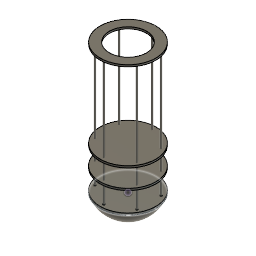
cansat+body (Autodesk Fusion 360 archive; units mm, degrees)
design "cansat body"
Autodesk Fusion 360 part; units mm, degrees
sketch "Sketch1" plane through (0, 0, 0) normal (0, 1, 0) x (1, 0, 0)
  circle A0 centre (0, 0) radius 75
  dimension "d1" = 150
  constraint coincident A0.centre origin
  measures "d1" diameter of A0
extrude "Extrude1" add sketch "Sketch1" along normal blind 5 makes body 1
sketch "Sketch2" plane through (0, 5, 0) normal (0, 1, 0) x (-1, 0, 0)
  circle A0 centre (0, 0) radius 75
  circle A1 centre (0.0043, -65) radius 2.5
  circle A2 centre (56.2938, -32.4963) radius 2.5
  circle A3 centre (56.2895, 32.5037) radius 2.5
  circle A4 centre (-56.2895, -32.5037) radius 2.5
  circle A5 centre (-0.0043, 65) radius 2.5
  circle A6 centre (-56.2938, 32.4963) radius 2.5
  dimension "d4" = 65
  dimension "d5" = 5
  dimension "d6" = 5
  dimension "d7" = 5
  dimension "d8" = 5
  dimension "d9" = 5
  dimension "d10" = 5
  constraint coincident A0.centre origin
  measures "d4" distance of A0.centre A5.centre
  measures "d5" diameter of A1
  measures "d6" diameter of A2
  measures "d7" diameter of A3
  measures "d8" diameter of A4
  measures "d9" diameter of A5
  measures "d10" diameter of A6
extrude "Extrude2" add sketch "Sketch2" along normal blind 350 contours A1 | A2 | A3 | A4 | A5 | A6 bodies 1
ref_plane "WorkPlane1" through (0, 355, 0) normal (0, 1, 0) x (1, 0, 0)
sketch "Sketch3" plane through (0, 355, 0) normal (0, 1, 0) x (1, 0, 0)
  circle A0 centre (0, 0) radius 75
  dimension "d14" = 150
  constraint coincident A0.centre origin
  measures "d14" diameter of A0
extrude "Extrude3" cut sketch "Sketch3" against normal blind 5 bodies 1
extrude "Extrude4" add sketch "Sketch3" against normal blind 5 from surface at -5 bodies 1
sketch "Sketch4" plane through (0, 350, 0) normal (0, 1, 0) x (-1, 0, 0)
  circle A0 centre (0, 0) radius 75
  circle A1 centre (0, 0) radius 50
  dimension "d19" = 100
  constraint coincident A0.centre A1.centre
  measures "d19" diameter of A1
extrude "Extrude5" cut sketch "Sketch4" against normal blind 5 contours A1 bodies 1
ref_plane "WorkPlane2" through (0, 110, 0) normal (0, 1, 0) x (1, 0, 0)
ref_plane "WorkPlane3" through (0, 57.5, 0) normal (0, 1, 0) x (1, 0, 0)
sketch "Sketch5" plane through (0, 110, 0) normal (0, 1, 0) x (1, 0, 0)
  circle A0 centre (0, 0) radius 75
  dimension "d24" = 150
  constraint coincident A0.centre origin
  measures "d24" diameter of A0
sketch "Sketch6" plane through (0, 57.5, 0) normal (0, 1, 0) x (1, 0, 0)
  circle A0 centre (0, 0) radius 75
  dimension "d25" = 150
  constraint coincident A0.centre origin
  measures "d25" diameter of A0
extrude "Extrude6" add sketch "Sketch5" along normal blind 5 separate body makes body 2
extrude "Extrude7" add sketch "Sketch6" along normal blind 5 separate body makes body 3
ref_plane "WorkPlane4" through (0, 2.5, 0) normal (0, 0, 1) x (0, 1, 0)
sketch "Sketch7" plane through (0, 0, 0) normal (0, 0, 1) x (1, 0, 0)
  line L0 (0, 0) -> (0, -50)
  arc A0 (0, -50) -> (75, 0) centre (3.5, 26) ccw
  line L1 (0, 0) -> (75, 0)
  dimension "d31" = 50
  constraint coincident L0.start L1.start
  constraint vertical L0
  constraint perpendicular L0 L1
  measures "d31" distance of L0.start L0.end
revolve "Revolve1" add sketch "Sketch7" angle 360 about axis through (0, 0, 0) along (0, -1, 0) bodies 1

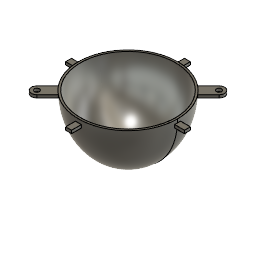
design "parachute container"
Autodesk Fusion 360 part; units mm, degrees
sketch "Sketch1" plane through (0, 0, 0) normal (0, 0, 1) x (1, 0, 0)
  line L0 (48, 0) -> (50, 0)
  ellipse E0 centre (0, 0) end of major axis (0, -60) minor radius 50 (0, -60) -> (50, 0) ccw
  line L1 (0, 0) -> (0, -38) construction
  spline S0 degree 3 poles (0, -58) (7.8191, -58) (15.6371, -55.6479) (22.5715, -51.1795) (29.3821, -46.7908) (35.3239, -40.3623) (39.6928, -32.5994) (44.1366, -24.7033) (46.9393, -15.4428) (47.7489, -5.9208) (47.9162, -3.9542) (48, -1.9771) (48, 0) knots 0 0 0 0 0.492802 0.492802 0.492802 0.976806 0.976806 0.976806 1.469118 1.469118 1.469118 1.570796 1.570796 1.570796 1.570796
  line L2 (0, -58) -> (0, -60)
  line L3 (0, -61.952) -> (0, -64)
  line L4 (0, -66) -> (2, -66)
  line L5 (2, -66) -> (2, -59.952)
  line L6 (0, -60) -> (-4, -60)
  line L7 (-4, -60) -> (-4, -66)
  line L8 (-4, -66) -> (0, -66)
  line L9 (-2, -61.952) -> (-2, -64)
  line L10 (-2, -61.952) -> (0, -61.952)
  line L11 (-2, -64) -> (0, -64)
  dimension "d1" = 120
  dimension "d2" = 100
  dimension "d12" = 6
  dimension "d13" = 2
  dimension "d14" = 4
  dimension "d16" = 2
  dimension "d18" = 2
  constraint coincident E0.centre L1.start
  constraint vertical L2
  constraint parallel L2 L3
  constraint perpendicular L3 L4
  constraint perpendicular L4 L5
  constraint coincident E0 L5.end
  constraint tangent E0 L6
  constraint perpendicular L2 L6
  constraint perpendicular L6 L7
  constraint perpendicular L8 L9
  constraint perpendicular L5 L10
  constraint perpendicular L5 L11
  measures "d1" distance of E0
  measures "d12" distance of L2.end L4.start
  measures "d13" distance of L4.start L4.end
  measures "d14" distance of L2.end L6.end
  measures "d16" distance of L7 L9
  measures "d18" distance of L4 L11
revolve "Revolve2" add sketch "Sketch1" angle 360 about axis through (0, 1.75, 0) along (0, 1, 0) contours L0 E0 S0 L2 makes body 1
extrude "Extrude1" add sketch "Sketch1" along normal mid plane 4 separate body contours E0 L4 L5 L6 L7 L8 makes body 2
sketch "Sketch2" plane through (0, 0, 0) normal (0, 0, 1) x (1, 0, 0)
  line L0 (3, -6.5) -> (-3, -6.5)
  line L1 (-3, -6.5) -> (-3, -3.5)
  line L2 (-3, -3.5) -> (3, -3.5)
  line L3 (3, -3.5) -> (3, -6.5)
  line L4 (3, -6.5) -> (-3, -3.5) construction
  line L5 (-3, -6.5) -> (3, -3.5) construction
  point P0 (0, -5)
  dimension "d40" = 6
  dimension "d41" = 3
  dimension "d42" = 5
  constraint horizontal L0
  constraint perpendicular L0 L1
  constraint parallel L0 L2
  constraint parallel L1 L3
  constraint coincident L4 P0
  constraint coincident L5 P0
  measures "d40" distance of L1.end L2.end
  measures "d41" distance of L0.end L1.end
  measures "d42" distance of origin P0
extrude "Extrude2" add sketch "Sketch2" along normal blind 10 from surface at 50 separate body makes body 3
pattern_circular "C-Pattern1" count 4 over 360 about axis through (0, 1.75, 0) along (0, 1, 0) of "Extrude2" makes body 4 at (53.3333, -6.5, -1) makes body 5 at (-1, -6.5, -53.3333) makes body 6 at (-53.3333, -6.5, 1)
sketch "Sketch3" plane through (0, 0, 0) normal (0, 1, 0) x (1, 0, 0)
  line L0 (0, 0) -> (57.0088, 0) construction
  circle A0 centre (45.9619, 45.9619) radius 2.55
  arc A1 (39.0613, 31.2124) -> (31.1808, 39.0865) centre (0, 0) ccw
  line L1 (42.0478, 49.8967) -> (31.1808, 39.0865)
  line L2 (49.8864, 42.0375) -> (39.0613, 31.2124)
  arc A2 (49.8864, 42.0375) -> (42.0478, 49.8967) centre (45.9619, 45.9619) ccw
  line L3 (0, 0) -> (-42.4264, 42.4264) construction
  line L4 (0, 0) -> (60, 0) construction
  line L5 (-49.8967, -42.0478) -> (-39.0865, -31.1808)
  arc A3 (-39.0865, -31.1808) -> (-31.2124, -39.0613) centre (0, 0) ccw
  line L6 (-42.0375, -49.8864) -> (-31.2124, -39.0613)
  circle A4 centre (-45.9619, -45.9619) radius 2.55
  arc A5 (-49.8967, -42.0478) -> (-42.0375, -49.8864) centre (-45.9619, -45.9619) ccw
  dimension "d29" = 65
  dimension "d30" = 5.1
  dimension "d31" = 100
  dimension "d36" = 135
  constraint horizontal L0
  constraint coincident L0.start A1.centre
  constraint concentric A0 A2
  constraint horizontal L4
  constraint symmetric A0 L3 A4
  constraint symmetric A1 L3 A3
  constraint symmetric L1.start L3 L5.start
  constraint symmetric L2.start L3 L6.start
  constraint symmetric A1.end L3 L5.end
  constraint symmetric A1.start L3 A3.end
  constraint symmetric A2 L3 A5
  measures "d29" distance of L0.start A0.centre
  measures "d30" diameter of A0
  measures "d31" diameter of A1
  measures "d36" angle of L3 L4
extrude "Extrude3" add sketch "Sketch3" against normal blind 3 bodies 1 2

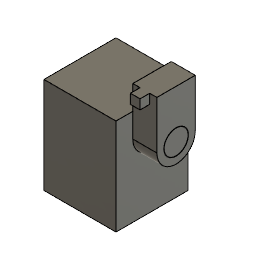
design "motor"
Autodesk Fusion 360 part; units mm, degrees
sketch "Sketch1" plane through (0, 0, 0) normal (0, 1, 0) x (1, 0, 0)
  line L0 (7.5, 7.5) -> (-7.5, 7.5)
  line L1 (-7.5, 7.5) -> (-7.5, -7.5)
  line L2 (-7.5, -7.5) -> (7.5, -7.5)
  line L3 (7.5, -7.5) -> (7.5, 7.5)
  line L4 (7.5, 7.5) -> (-7.5, -7.5) construction
  line L5 (-7.5, 7.5) -> (7.5, -7.5) construction
  dimension "d1" = 15
  dimension "d2" = 15
  constraint horizontal L0
  constraint perpendicular L0 L1
  constraint parallel L0 L2
  constraint parallel L1 L3
  constraint coincident L4 origin
  constraint coincident L5 origin
  measures "d1" distance of L1.end L2.end
  measures "d2" distance of L0.end L1.end
extrude "Extrude1" add sketch "Sketch1" along normal blind 20
sketch "Sketch2" plane through (7.5, 0, 0) normal (1, 0, 0) x (0, 0, -1)
  line L0 (-7.5, 0) -> (7.5, 0)
  line L1 (7.5, 0) -> (7.5, 20)
  line L2 (7.5, 20) -> (-7.5, 20)
  line L3 (-7.5, 20) -> (-7.5, 0)
  circle A0 centre (0, 15) radius 2.5
  dimension "d5" = 5
  measures "d5" diameter of A0
extrude "Extrude2" add sketch "Sketch2" along normal blind 5 contours A0
sketch "Sketch3" plane through (7.5, 0, 0) normal (1, 0, 0) x (0, 0, -1)
  circle A0 centre (0, 15) radius 2.5
  line L0 (-7.5, 0) -> (7.5, 0)
  line L1 (7.5, 0) -> (7.5, 20)
  line L2 (7.5, 20) -> (-7.5, 20)
  line L3 (-7.5, 20) -> (-7.5, 0)
  circle A1 centre (0, 15) radius 2.55
  line L4 (-4, 15) -> (-4, 25)
  line L5 (4, 15) -> (4, 25)
  arc A2 (-4, 15) -> (4, 15) centre (0, 15) ccw
  line L6 (-4, 25) -> (4, 25)
  dimension "d8" = 5.1
  dimension "d9" = 8
  dimension "d10" = 10
  dimension "d11" = 10
  constraint concentric A0 A1
  constraint concentric A1 A2
  constraint vertical L4
  constraint tangent L4 A2
  constraint perpendicular L2 L5
  constraint tangent L5 A2
  measures "d8" diameter of A1
  measures "d9" diameter of A2
  measures "d10" distance of L4.start L4.end
  measures "d11" distance of L5.start L5.end
extrude "Extrude3" add sketch "Sketch3" along normal blind 5 contours L2 L4 L5 L6 | L2 L4 L5 A2
sketch "Sketch4" plane through (0, 0, 4) normal (0, 0, 1) x (1, 0, 0)
  line L0 (7.5, 20) -> (7.5, 15)
  line L1 (7.5, 15) -> (12.5, 15)
  line L2 (12.5, 15) -> (12.5, 25)
  line L3 (12.5, 25) -> (7.5, 25)
  line L4 (7.5, 25) -> (7.5, 20)
  line L5 (9, 25) -> (11, 25)
  line L6 (11, 25) -> (11, 23)
  line L7 (9, 25) -> (9, 23)
  line L8 (9, 23) -> (11, 23)
  point P0 (10, 25)
  dimension "d14" = 2
  dimension "d15" = 2
  dimension "d16" = 2
  constraint midpoint L5 P0
  constraint coincident L3 P0
  constraint perpendicular L4 L5
  constraint perpendicular L5 L6
  constraint perpendicular L5 L7
  measures "d14" distance of L5.start L5.end
  measures "d15" distance of L5.end L6.end
  measures "d16" distance of L5.start L7.end
extrude "Extrude4" add sketch "Sketch4" along normal blind 2 contours L3 L5 L6 L7 L8
